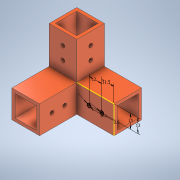
# Autodesk Inventor part: esquina20mm
Saved by Autodesk Inventor 2022.6 (Build 266554000, 554)
## iProperties
Created: 2024-09-02
Part Number: esquina20mm
Material: Genérico
Document SubType Name: Modeling
Designer: G207
Density: 1 g/cm^3
Appearance: Valor por defecto
Author: G207
Autodesk Inventor part; units mm, degrees
ref_plane "YZ Plane" through (0, 0, 0) normal (1, 0, 0) x (0, 1, 0)
ref_plane "XZ Plane" through (0, 0, 0) normal (0, 1, 0) x (-1, 0, 0)
ref_plane "XY Plane" through (0, 0, 0) normal (0, 0, 1) x (1, 0, 0)
sketch "Boceto1" plane through (0, 0, 0) normal (0, 0, 1) x (1, 0, 0)
  line L0 (0, 0) -> (50, 0)
  line L1 (50, 0) -> (50, 26)
  line L2 (50, 26) -> (26, 26)
  line L3 (0, 26) -> (0, 0)
  line L4 (0, 0) -> (26, 0)
  line L5 (26, 26) -> (26, 50)
  line L6 (26, 50) -> (0, 50)
  line L7 (0, 50) -> (0, 0)
  line L8 (0, 0) -> (50, 0)
  line L9 (50, 0) -> (50, 3)
  line L10 (50, 3) -> (0, 3)
  line L11 (0, 3) -> (0, 0)
  line L12 (0, 50) -> (3, 50)
  line L13 (3, 50) -> (3, 0)
  line L14 (3, 0) -> (0, 0)
  line L15 (0, 0) -> (0, 50)
  line L16 (26, 50) -> (23, 50)
  line L17 (23, 50) -> (23, 24)
  line L18 (23, 24) -> (26, 24)
  line L19 (26, 24) -> (26, 50)
  line L20 (50, 26) -> (23, 26)
  line L21 (23, 26) -> (23, 23)
  line L22 (23, 23) -> (50, 23)
  line L23 (50, 23) -> (50, 26)
  line L24 (23, 50) -> (1.5, 50)
  line L25 (3, 3) -> (50, 3)
  line L26 (50, 23) -> (23, 23)
  point P0 (3, 3)
  dimension "d0" = 50
  dimension "d1" = 26
  dimension "d2" = 26
  dimension "d3" = 50
  dimension "d4" = 50
  dimension "d5" = 3
  dimension "d6" = 3
  dimension "d7" = 50
  dimension "d8" = 3
  dimension "d9" = 26
  dimension "d10" = 27
  dimension "d11" = 3
  constraints: 54 end point, 13 parallel, 6 horizontal, 6 perpendicular, 2 point on line, 1 collinear, 1 midpoint
  measures "d0" distance of L3.start L1.end
  measures "d1" distance of L0.end L1.end
  measures "d2" distance of L6.end L5.end
  measures "d3" distance of L5.end L4.end
  measures "d4" distance of L10.end L9.end
  measures "d5" distance of L9.end L8.end
  measures "d6" distance of L13.end L14.end
  measures "d7" distance of L12.end L13.end
  measures "d8" distance of L18.end L17.end
  measures "d9" distance of L17.end L16.end
  measures "d10" distance of L22.end L21.end
  measures "d11" distance of L21.end L20.end
extrude "Extrusión1" add sketch "Boceto1" along normal blind 26 contours L3 L10 L13 L0 | L13 L10 L1 L0
extrude "Extrusión2" add sketch "Boceto1" along normal blind 26 contours L3 L7 L6 L13 L10
extrude "Extrusión3" add sketch "Boceto1" along normal blind 26 contours L22 L21 L18 L19 L2 L1 | L20 L19 L18 L17
extrude "Extrusión4" add sketch "Boceto1" along normal blind 26 contours L6 L5 L20 L17
sketch "Boceto2" plane through (0, 0, 26) normal (0, 0, 1) x (1, 0, 0)
  line L0 (3, 50) -> (0, 50) projected
  line L1 (26, 50) -> (23, 50) projected
  line L2 (0, 50) -> (26, 50)
  line L3 (3, 50) -> (23, 50)
  line L4 (23, 50) -> (23, 23) projected
  line L5 (23, 23) -> (50, 23) projected
  line L6 (23, 23) -> (50, 23)
  line L7 (50, 0) -> (50, 3) projected
  line L8 (50, 23) -> (50, 3)
  line L9 (50, 3) -> (3, 3) projected
  line L10 (50, 3) -> (3, 3)
  line L11 (3, 3) -> (3, 50)
  point P0 (0, 0)
  constraints: 12 end point, 2 collinear, 2 horizontal, 2 perpendicular
extrude "Extrusión5" add sketch "Boceto2" against normal blind 3
extrude "Extrusión6" add sketch "Boceto1" along normal blind 3 contours L13 L6 L17 L21 L22 L1 L10
sketch "Boceto3" plane through (0, 0, 26) normal (0, 0, 1) x (1, 0, 0)
  line L0 (0, 0) -> (50, 0) projected
  line L1 (0, 0) -> (26, 0)
  line L2 (0, 0) -> (26, 0) construction
  line L3 (50, 26) -> (26, 26) projected
  line L4 (26, 0) -> (26, 26)
  line L5 (26, 26) -> (0, 26)
  line L6 (3, 3) -> (3, 50) projected
  line L7 (0, 26) -> (0, 0)
  line L8 (3, 3) -> (50, 3) projected
  line L9 (3, 3) -> (23, 3)
  line L10 (23, 3) -> (23, 23)
  line L11 (23, 23) -> (3, 23)
  line L12 (3, 23) -> (3, 3)
  dimension "d24" = 26
  dimension "d25" = 0
  dimension "d26" = 20
  dimension "d27" = 20
  constraints: 18 end point, 3 perpendicular, 2 collinear, 2 horizontal, 2 parallel
  measures "d24" distance of L0.start L1.end
  measures "d25" distance between parallel lines of L1 L2
  measures "d26" distance of L11.end L10.end
  measures "d27" distance of L10.end L9.end
extrude "Extrusión7" cut sketch "Boceto3" against normal blind 3 contours L8 L6 L11 L10
sketch "Boceto4" plane through (0, 0, 26) normal (0, 0, 1) x (1, 0, 0)
  line L0 (0, 0) -> (26, 0)
  line L1 (0, 0) -> (50, 0) projected
  line L2 (0, 0) -> (26, 0) construction
  line L3 (26, 0) -> (26, 26)
  line L4 (26, 26) -> (0, 26)
  line L5 (3, 23) -> (23, 23) projected
  line L6 (0, 50) -> (0, 0) projected
  line L7 (0, 26) -> (0, 0)
  line L8 (50, 23) -> (23, 23) projected
  line L9 (3, 23) -> (23, 23)
  line L10 (23, 23) -> (23, 3) projected
  line L11 (23, 23) -> (23, 3)
  line L12 (50, 3) -> (3, 3) projected
  line L13 (23, 3) -> (3, 3)
  line L14 (3, 3) -> (3, 23)
  dimension "d30" = 26
  dimension "d31" = 0
  dimension "d32" = 26
  dimension "d33" = 90
  constraints: 18 end point, 4 perpendicular, 3 collinear, 2 horizontal, 1 parallel
  measures "d30" distance of L0.start L0.end
  measures "d31" distance between parallel lines of L0 L2
  measures "d32" distance of L0.end L3.end
  measures "d33" angle of L3 L0
extrude "Extrusión8" add sketch "Boceto4" along normal blind 35 contours L6 L4 L3 L8 L5 L14 L12 L0 | L12 L10 L8 L3
sketch "Boceto5" plane through (26, 0, 26) normal (1, 0, 0) x (0, 0, -1)
  circle A0 centre (-23.5, 13) radius 1.75
  circle A1 centre (-11.5, 13) radius 1.75
  line L0 (0, 26) -> (-35, 26) projected
  line L1 (-35, 0) -> (-35, 26) projected
  line L2 (0, 0) -> (0, 26) projected
  point P0 (26, 0)
  dimension "d36" = 3.5
  dimension "d37" = 3.5
  dimension "d38" = 13
  dimension "d39" = 13
  dimension "d40" = 12
  dimension "d41" = 11.5
  dimension "d42" = 35
  dimension "d43" = 11.5
  constraints: 2 centre point
  measures "d36" diameter of A0
  measures "d37" diameter of A1
  measures "d38" distance from line of L0 A0.centre
  measures "d39" distance from line of L0 A1.centre
  measures "d40" distance of A1.centre A0.centre
  measures "d41" distance from line of L1 A0.centre
  measures "d42" distance between parallel lines of L2 L1
  measures "d43" distance from line of L2 A1.centre
sketch "Boceto6" plane through (50, 0, 26) normal (1, 0, 0) x (0, 0, -1)
  line L0 (26, 26) -> (0, 26) projected
  line L1 (26, 26) -> (26, 50) projected
  line L2 (0, 26) -> (26, 26)
  line L3 (26, 50) -> (26, 0) projected
  line L4 (26, 26) -> (26, 0)
  line L5 (26, 0) -> (0, 0)
  line L6 (26, 0) -> (-35, 0) projected
  line L7 (23, 23) -> (3, 23) projected
  line L8 (3, 23) -> (23, 23)
  line L9 (23, 23) -> (23, 3)
  line L10 (23, 3) -> (3, 3)
  line L11 (23, 3) -> (-35, 3) projected
  line L12 (-35, 23) -> (3, 23) projected
  line L13 (3, 3) -> (3, 23)
  line L14 (0, 26) -> (0, 0)
  constraints: 16 end point, 4 perpendicular, 2 horizontal, 2 point on line
extrude "Extrusión9" add sketch "Boceto6" along normal blind 11 contours L3 L5 L14 L11 L10 L9 L7 L12 L0 | L12 L13 L11 L14
sketch "Boceto7" plane through (0, 50, 26) normal (0, 1, 0) x (1, 0, 0)
  line L0 (3, 3) -> (23, 3) projected
  line L1 (3, 3) -> (23, 3)
  line L2 (23, 3) -> (23, 23)
  line L3 (23, 23) -> (3, 23)
  line L4 (3, 23) -> (3, 3)
  line L5 (26, 26) -> (26, 0) projected
  line L6 (26, 26) -> (0, 26)
  line L7 (0, 26) -> (0, 0)
  line L8 (0, 0) -> (26, 0)
  line L9 (26, 0) -> (26, 26)
  dimension "d46" = 20
  dimension "d47" = 20
  dimension "d48" = 26
  dimension "d49" = 26
  constraints: 16 end point, 4 parallel, 2 horizontal, 2 perpendicular
  measures "d46" distance of L3.end L2.end
  measures "d47" distance of L2.end L1.end
  measures "d48" distance of L8.end L7.end
  measures "d49" distance of L7.end L6.end
extrude "Extrusión10" add sketch "Boceto7" along normal blind 11
sketch "Boceto8" plane through (0, 0, 26) normal (0, 0, 1) x (1, 0, 0)
  circle A0 centre (49.5, 13) radius 1.75
  circle A1 centre (37.5, 13) radius 1.75
  line L0 (61, 26) -> (61, 0) projected
  line L1 (26, 26) -> (61, 26) projected
  point P0 (0, 0)
  dimension "d52" = 3.5
  dimension "d53" = 3.5
  dimension "d54" = 11.5
  dimension "d55" = 12
  dimension "d56" = 13
  dimension "d57" = 13
  constraints: 2 centre point
  measures "d52" diameter of A0
  measures "d53" diameter of A1
  measures "d54" distance from line of L0 A0.centre
  measures "d55" distance of A0.centre A1.centre
  measures "d56" distance from line of L1 A0.centre
  measures "d57" distance from line of L1 A1.centre
extrude "Extrusión11" cut sketch "Boceto5" against normal up to next contours A0
extrude "Extrusión12" cut sketch "Boceto5" against normal up to next contours A1
extrude "Extrusión13" cut sketch "Boceto8" against normal up to next contours A1
extrude "Extrusión14" cut sketch "Boceto8" against normal up to next contours A0
sketch "Boceto9" plane through (0, 0, 26) normal (0, 0, 1) x (1, 0, 0)
  circle A0 centre (13, 37.5) radius 1.75
  circle A1 centre (13, 49.5) radius 1.75
  line L0 (0, 26) -> (0, 61) projected
  line L1 (0, 61) -> (26, 61) projected
  point P0 (0, 0)
  dimension "d66" = 3.5
  dimension "d67" = 3.5
  dimension "d68" = 13
  dimension "d69" = 13
  dimension "d70" = 11.5
  dimension "d71" = 12
  constraints: 2 centre point
  measures "d66" diameter of A0
  measures "d67" diameter of A1
  measures "d68" distance from line of L0 A0.centre
  measures "d69" distance from line of L0 A1.centre
  measures "d70" distance from line of L1 A1.centre
  measures "d71" distance of A1.centre A0.centre
sketch "Boceto10" plane through (26, 26, 26) normal (1, 0, 0) x (0, 0, -1)
  circle A0 centre (13, 23.5) radius 1.75
  circle A1 centre (13, 11.5) radius 1.75
  line L0 (0, 0) -> (0, 35) projected
  line L1 (0, 35) -> (26, 35) projected
  point P0 (26, -26)
  dimension "d72" = 3.5
  dimension "d73" = 3.5
  dimension "d74" = 13
  dimension "d75" = 13
  dimension "d76" = 12
  dimension "d77" = 11.5
  constraints: 2 centre point
  measures "d72" diameter of A0
  measures "d73" diameter of A1
  measures "d74" distance from line of L0 A0.centre
  measures "d75" distance from line of L0 A1.centre
  measures "d76" distance of A1.centre A0.centre
  measures "d77" distance from line of L1 A0.centre
extrude "Extrusión15" cut sketch "Boceto9" against normal up to next contours A1
extrude "Extrusión16" cut sketch "Boceto9" against normal up to next contours A0
extrude "Extrusión17" cut sketch "Boceto10" against normal up to next contours A0
extrude "Extrusión18" cut sketch "Boceto10" against normal up to next contours A1
